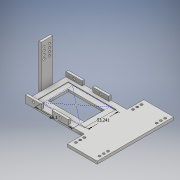
# Autodesk Inventor part: LIner
Saved by Autodesk Inventor 2018.1 (Build 221171000, 171)
## iProperties
Created: 2019-02-17
Part Number: LIner
Material: Типовые
Document SubType Name: Modeling
Designer: kostya
Density: 1 g/cm^3
Appearance: По умолчанию
Author: kostya
Autodesk Inventor part; units mm, degrees
ref_plane "YZ Plane" through (0, 0, 0) normal (1, 0, 0) x (0, 1, 0)
ref_plane "XZ Plane" through (0, 0, 0) normal (0, 1, 0) x (-1, 0, 0)
ref_plane "XY Plane" through (0, 0, 0) normal (0, 0, 1) x (1, 0, 0)
sketch "Эскиз1" plane through (0, 0, 0) normal (0, 0, 1) x (1, 0, 0)
  line L0 (-42.5, -28.25) -> (42.5, -28.25) construction
  line L1 (42.5, -28.25) -> (42.5, 28.25) construction
  line L2 (42.5, 28.25) -> (-42.5, 28.25) construction
  line L3 (-42.5, 28.25) -> (-42.5, -28.25) construction
  line L4 (-52.25, 38) -> (52.25, 38)
  line L5 (52.25, 38) -> (52.25, -38)
  line L6 (52.25, -38) -> (-52.25, -38)
  line L7 (-52.25, -38) -> (-52.25, 38)
  line L8 (52.25, 38) -> (52.25, 68) construction
  line L9 (52.25, 68) -> (105.25, 68) construction
  line L10 (105.25, 68) -> (105.25, 0) construction
  line L11 (105.25, 0) -> (105.25, -68) construction
  line L12 (105.25, -68) -> (52.25, -68) construction
  line L13 (52.25, -68) -> (52.25, 0) construction
  line L14 (52.25, 38) -> (52.25, 68)
  line L15 (105.25, 68) -> (52.25, 68)
  line L16 (105.25, 68) -> (105.25, -68)
  line L17 (105.25, -68) -> (52.25, -68)
  line L18 (52.25, -68) -> (52.25, 0)
  line L19 (-42.5, -28.25) -> (42.5, -28.25)
  line L20 (42.5, 28.25) -> (42.5, -28.25)
  line L21 (-42.5, -28.25) -> (-42.5, 28.25)
  line L22 (42.5, 28.25) -> (-42.5, 28.25)
  dimension "d0" = 85
  dimension "d1" = 56.5
  dimension "d2" = 9.75
  dimension "d3" = 68
  dimension "d4" = 53
  dimension "d5" = 68
  constraints: 46 end point, 7 collinear, 7 perpendicular, 4 parallel, 2 horizontal, 2 vertical, 1 midpoint, 3 other
  measures "d0" distance of L2.end L1.end
  measures "d1" distance of L1.end L0.end
  measures "d2" distance between parallel lines of L2 L4
  measures "d3" distance of L13.end L8.end
  measures "d4" distance of L8.end L9.end
  measures "d5" distance of L10.end L11.end
extrude "Выдавливание1" add sketch "Эскиз1" along normal blind 5 contours L4 L5 L6 L7 | L14 L15 L16 L17 L18 L5 | L21 L22 L20 L19
sketch "Эскиз4" plane through (0, 0, 5) normal (0, 0, 1) x (1, 0, 0)
  line L0 (-42.5, -28.25) -> (42.5, -28.25) construction
  line L1 (-42.5, -28.25) -> (-42.5, 28.25) projected
  line L2 (42.5, 28.25) -> (-42.5, 28.25) construction
  line L3 (-42.5, 28.25) -> (42.5, 28.25)
  line L4 (42.5, 28.25) -> (42.5, -28.25)
  line L5 (42.5, -28.25) -> (-42.5, -28.25)
  line L6 (-42.5, -28.25) -> (-42.5, 28.25)
  point P0 (0, 0)
  constraints: 8 end point, 2 parallel, 1 horizontal, 1 perpendicular
extrude "Выдавливание3" cut sketch "Эскиз4" against normal blind 1
sketch "Эскиз5" plane through (0, 0, 4) normal (0, 0, 1) x (1, 0, 0)
  line L0 (42.5, 28.25) -> (42.5, -28.25) projected
  line L1 (-42.5, 28.25) -> (42.5, 28.25) projected
  line L2 (-42.5, -28.25) -> (-42.5, 28.25) projected
  line L3 (42.5, -28.25) -> (-42.5, -28.25) projected
  line L4 (32.25, 18) -> (32.25, -18)
  line L5 (32.25, -18) -> (-32.25, -18)
  line L6 (-32.25, -18) -> (-32.25, 18)
  line L7 (-32.25, 18) -> (32.25, 18)
  point P0 (0, 0)
  dimension "d12" = 10.25
  constraints: 8 end point, 3 other
  measures "d12" distance between parallel lines of L1 L7
extrude "Выдавливание4" cut sketch "Эскиз5" against normal blind 8 contours L4 L5 L6 L7
sketch "Эскиз6" plane through (0, 0, 5) normal (0, 0, 1) x (1, 0, 0)
  line L0 (-33.05, 26.6205) -> (33.05, 26.6205) construction
  line L1 (33.05, 26.6205) -> (33.05, -26.6205) construction
  line L2 (33.05, -26.6205) -> (-33.05, -26.6205) construction
  line L3 (-33.05, -26.6205) -> (-33.05, 26.6205) construction
  line L4 (-33.05, 26.6205) -> (33.05, -26.6205) construction
  line L5 (33.05, 26.6205) -> (-33.05, -26.6205) construction
  point P0 (0, 0)
  dimension "d15" = 66.1
  dimension "d16" = 53.241
  constraints: 12 end point, 2 midpoint, 2 parallel, 1 horizontal, 1 perpendicular
  measures "d15" distance of L1.end L2.end
  measures "d16" distance of L0.end L1.end
sketch "Эскиз7" plane through (0, 0, 5) normal (0, 0, 1) x (1, 0, 0)
  line L0 (-52.25, 38) -> (-52.25, -38) construction
  line L1 (-52.25, 0) -> (-56.25, 0)
  line L2 (-56.25, 10) -> (-52.25, 10)
  line L3 (-52.25, 10) -> (-52.25, -10)
  line L4 (-52.25, -10) -> (-56.25, -10)
  line L5 (-56.25, -10) -> (-56.25, 10)
  line L6 (-56.25, 10) -> (-52.25, -10) construction
  line L7 (-52.25, 10) -> (-56.25, -10) construction
  point P0 (0, 0)
  point P1 (-54.25, 0)
  dimension "d17" = 4
  dimension "d18" = 20
  constraints: 14 end point, 4 midpoint, 2 horizontal, 2 parallel, 1 perpendicular, 1 point on line
  measures "d17" distance of L1.start L1.end
  measures "d18" distance of L2.end L3.end
extrude "Выдавливание5" add sketch "Эскиз7" along normal blind 75 and the other way blind 5
sketch "Эскиз8" plane through (-56.25, -10, 80) normal (-1, 0, 0) x (0, 0, 1)
  line L0 (0, 0) -> (-80, 0) projected
  line L1 (0, 20) -> (0, 0) projected
  line L2 (-80, 20) -> (0, 20) projected
  line L3 (-80, 0) -> (-80, 20) projected
  line L4 (-80, 0) -> (-33.989, 0) construction
  line L5 (0, 0) -> (-80, 0) construction
  line L6 (-33.989, 0) -> (-33.989, 20) construction
  line L7 (0, 20) -> (-75, 20) construction
  line L8 (-33.989, 20) -> (-27.805, 20) construction
  line L9 (-27.805, 20) -> (-27.805, 14.454) construction
  circle A0 centre (-27.805, 14.454) radius 2
  line L10 (-27.805, 14.454) -> (-21.488, 14.454) construction
  line L11 (-27.805, 14.454) -> (-27.805, 5) construction
  circle A1 centre (-27.805, 5) radius 2
  circle A2 centre (-21.488, 14.454) radius 2
  circle A3 centre (-21.488, 5) radius 2
  circle A4 centre (-15.171, 14.454) radius 2
  circle A5 centre (-15.171, 5) radius 2
  circle A6 centre (-8.854, 14.454) radius 2
  circle A7 centre (-8.854, 5) radius 2
  point P0 (-80, 10)
  dimension "d23" = 46.011
  dimension "d24" = 6.184
  dimension "d25" = 5.546
  dimension "d26" = 4
  dimension "d27" = 6.317
  dimension "d28" = 9.454
  dimension "d29" = 4
  dimension "d32" = 6.317
  constraints: 12 end point, 8 centre point, 3 point on line, 2 coincident, 2 horizontal, 2 vertical, 1 perpendicular, 12 other
  measures "d23" distance of L0.end L4.end
  measures "d24" distance of L6.end L8.end
  measures "d25" distance of L8.end L9.end
  measures "d26" diameter of A0
  measures "d27" distance of L10.start L10.end
  measures "d28" distance of L10.start L11.end
  measures "d29" diameter of A1
  measures "d32" distance of L10.start A2.centre
extrude "Выдавливание6" cut sketch "Эскиз8" against normal blind 75 contours A0 | A1 | A2 | A3 | A4 | A5 | A6 | A7
sketch "Эскиз9" plane through (0, 0, 0) normal (0, 0, -1) x (-1, 0, 0)
  line L0 (-32.25, 18) -> (32.25, 18) projected
  line L1 (32.25, 18) -> (32.25, -18) projected
  line L2 (32.25, -18) -> (-32.25, -18) projected
  line L3 (-32.25, -18) -> (-32.25, 18) projected
  line L4 (-52.25, 68) -> (-52.25, 38) projected
  line L5 (-105.25, 68) -> (-52.25, 68) projected
  line L6 (-105.25, -68) -> (-105.25, 68) projected
  line L7 (-52.25, -68) -> (-105.25, -68) projected
  line L8 (-52.25, -38) -> (-52.25, -68) projected
  line L9 (52.25, -38) -> (-52.25, -38) projected
  line L10 (52.25, -10) -> (52.25, -38) projected
  line L11 (52.25, -10) -> (56.25, -10) projected
  line L12 (56.25, -10) -> (56.25, 10) projected
  line L13 (56.25, 10) -> (52.25, 10) projected
  line L14 (52.25, 38) -> (52.25, 10) projected
  line L15 (-52.25, 38) -> (52.25, 38) projected
  line L16 (52.25, -38) -> (52.25, -42) construction
  line L17 (52.25, -38) -> (-52.25, -38) projected
  line L18 (52.25, -38) -> (23.7, -38)
  line L19 (4.7, -38) -> (-23.85, -38)
  line L20 (56.25, 0) -> (0, 0) construction
  line L21 (52.25, 38) -> (-52.25, 38)
  line L22 (52.25, 38) -> (52.25, 42) construction
  line L23 (4.7, 38) -> (-23.85, 38)
  line L24 (23.7, 34) -> (52.25, 34)
  line L25 (23.7, 38) -> (23.7, 34)
  line L26 (52.25, 38) -> (52.25, 34) construction
  line L27 (52.25, 34) -> (52.25, 38)
  line L28 (4.7, 34) -> (4.7, 38)
  line L29 (-23.85, 34) -> (4.7, 34)
  line L30 (-23.85, 38) -> (-23.85, 34)
  line L31 (52.25, -38) -> (52.25, -34) construction
  line L32 (23.7, -38) -> (23.7, -34)
  line L33 (23.7, -34) -> (52.25, -34)
  line L34 (52.25, -34) -> (52.25, -38)
  line L35 (-23.85, -38) -> (-23.85, -34)
  line L36 (-23.85, -34) -> (4.7, -34)
  line L37 (4.7, -34) -> (4.7, -38)
  line L38 (52.25, 34) -> (23.7, 34)
  line L39 (23.7, 34) -> (23.7, 38)
  line L40 (23.7, 38) -> (52.25, 38)
  line L41 (52.25, 38) -> (52.25, 34)
  line L42 (4.7, 34) -> (-23.85, 34)
  line L43 (-23.85, 34) -> (-23.85, 38)
  line L44 (-23.85, 38) -> (4.7, 38)
  line L45 (4.7, 38) -> (4.7, 34)
  dimension "d39" = 4
  constraints: 58 end point, 6 symmetric about line, 5 horizontal, 4 parallel, 2 perpendicular, 1 midpoint, 1 point on line, 1 vertical
  measures "d39" distance of L9.start L16.end
extrude "Выдавливание7" add sketch "Эскиз9" against normal blind 13 contours L15 L28 L29 L30 | L15 L14 L24 L25 | L35 L36 L37 L9 | L32 L33 L10 L9
sketch "Эскиз10" plane through (-52.25, 38, 0) normal (0, 1, 0) x (1, 0, 0)
  line L0 (47.55, -5) -> (28.55, -5) construction
  line L1 (28.55, -5) -> (0, -5) construction
  line L2 (0, 0) -> (0, -13) construction
  line L3 (0, -5) -> (0, -13) construction
  line L4 (0, -13) -> (0, -5) construction
  circle A0 centre (14.275, -9) radius 2
  line L5 (38.05, -7) -> (38.05, -12) construction
  circle A1 centre (61.825, -9) radius 2
  point P0 (52.25, 0)
  dimension "d45" = 4
  constraints: 6 end point, 2 centre point, 1 collinear, 1 horizontal, 1 point on line, 1 symmetric about line, 1 vertical, 1 other
  measures "d45" diameter of A0
extrude "Выдавливание8" cut sketch "Эскиз10" against normal up to surface (76 mm away)
sketch "Эскиз11" plane through (0, 0, 5) normal (0, 0, 1) x (1, 0, 0)
  line L0 (-42.5, 28.25) -> (42.5, 28.25) projected
  line L1 (42.5, 28.25) -> (42.5, -28.25) projected
  line L2 (42.5, -28.25) -> (-42.5, -28.25) projected
  line L3 (-42.5, -28.25) -> (-42.5, 28.25) projected
  line L4 (-23.7, 38) -> (-23.7, 34) projected
  line L5 (-23.7, 34) -> (-52.25, 34) projected
  line L6 (-52.25, 34) -> (-52.25, 10) projected
  line L7 (-52.25, 10) -> (-52.25, -10) projected
  line L8 (-52.25, -10) -> (-52.25, -34) projected
  line L9 (-52.25, -34) -> (-23.7, -34) projected
  line L10 (-23.7, -34) -> (-23.7, -38) projected
  line L11 (-23.7, -38) -> (-4.7, -38) projected
  line L12 (-4.7, -38) -> (-4.7, -34) projected
  line L13 (-4.7, -34) -> (23.85, -34) projected
  line L14 (23.85, -34) -> (23.85, -38) projected
  line L15 (23.85, -38) -> (52.25, -38) projected
  line L16 (52.25, -38) -> (52.25, -68) projected
  line L17 (52.25, -68) -> (105.25, -68) projected
  line L18 (105.25, -68) -> (105.25, 68) projected
  line L19 (105.25, 68) -> (52.25, 68) projected
  line L20 (52.25, 68) -> (52.25, 38) projected
  line L21 (52.25, 38) -> (23.85, 38) projected
  line L22 (23.85, 38) -> (23.85, 34) projected
  line L23 (23.85, 34) -> (-4.7, 34) projected
  line L24 (-4.7, 34) -> (-4.7, 38) projected
  line L25 (-4.7, 38) -> (-23.7, 38) projected
  line L26 (52.25, -38) -> (52.25, -68) projected
  line L27 (52.25, -68) -> (57.75, -68)
  line L28 (52.25, -68) -> (105.25, -68) projected
  line L29 (57.75, -68) -> (57.75, -38) construction
  line L30 (23.85, -38) -> (52.25, -38) projected
  line L31 (57.75, -38) -> (52.25, -38) construction
  line L32 (57.75, -68) -> (57.75, -58.3)
  circle A0 centre (57.75, -58.3) radius 2
  line L33 (57.75, -58.3) -> (57.75, -50.8) construction
  circle A1 centre (57.75, -50.8) radius 2
  circle A2 centre (57.75, -43.3) radius 2
  line L34 (52.25, -68) -> (105.25, -68) construction
  line L35 (78.75, -68) -> (78.75, -28.25) construction
  circle A3 centre (99.75, -58.3) radius 2
  circle A4 centre (99.75, -50.8) radius 2
  circle A5 centre (99.75, -43.3) radius 2
  line L36 (105.25, -68) -> (105.25, 68) construction
  line L37 (105.25, 0) -> (77, 0) construction
  circle A6 centre (57.75, 58.3) radius 2
  circle A7 centre (57.75, 50.8) radius 2
  circle A8 centre (57.75, 43.3) radius 2
  circle A9 centre (99.75, 58.3) radius 2
  circle A10 centre (99.75, 50.8) radius 2
  circle A11 centre (99.75, 43.3) radius 2
  point P0 (0, 0)
  dimension "d48" = 5.5
  dimension "d49" = 9.7
  dimension "d50" = 4
  dimension "d51" = 7.5
  dimension "d54" = 7.5
  constraints: 14 end point, 12 centre point, 9 symmetric about line, 3 point on line, 2 midpoint, 2 perpendicular, 2 vertical, 1 coincident, 1 horizontal, 13 other
  measures "d48" distance of L16.end L27.end
  measures "d49" distance of L27.end L32.end
  measures "d50" diameter of A0
  measures "d51" distance of L33.start L33.end
  measures "d54" distance of L33.start A1.centre
extrude "Выдавливание9" cut sketch "Эскиз11" against normal blind 10 contours A0 | A1 | A2 | A3 | A4 | A5 | A6 | A7 | A8 | A9 | A10 | A11
